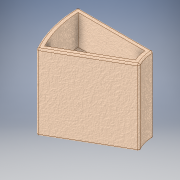
# Autodesk Inventor part: angular30
Saved by Autodesk Inventor 2019 (Build 230136000, 136)
## iProperties
Created: 2019-02-27
Part Number: angular30
Material: Concrete
Document SubType Name: Modeling
Designer: gaincarlo
Density: 2.40731 g/cm^3
Appearance: Exterior - Beige
Author: gaincarlo
Autodesk Inventor part; units mm, degrees
ref_plane "YZ Plane" through (0, 0, 0) normal (1, 0, 0) x (0, 1, 0)
ref_plane "XZ Plane" through (0, 0, 0) normal (0, 1, 0) x (-1, 0, 0)
ref_plane "XY Plane" through (0, 0, 0) normal (0, 0, 1) x (1, 0, 0)
sketch "Sketch1" plane through (0, 0, 0) normal (0, 1, 0) x (-1, 0, 0)
  line L0 (0, 0) -> (500, 0)
  arc A0 (500, 0) -> (399.5191, 375) centre (-250, 0) ccw
  arc A1 (0, 0) -> (-33.4936, 125) centre (-250, 0) ccw
  line L1 (-33.4936, 125) -> (399.5191, 375)
  line L2 (-404.937, 0) -> (679.6218, 0) projected
  dimension "d1" = 500
  dimension "d2" = 30
  dimension "d10" = 250
  constraints: 4 end point, 4 point on circle, 3 point on line, 2 centre point, 1 coincident, 1 horizontal
  measures "d1" distance of L0.start L0.end
  measures "d2" angle of L0 L1
  measures "d10" radius of A1
extrude "Extrusion1" add sketch "Sketch1" along normal blind 500
sketch "Sketch2" plane through (0, 500, 0) normal (0, 1, 0) x (1, 0, 0)
  arc A0 (0, 0) -> (33.4936, -125) centre (250, 0) ccw projected
  line L0 (33.4936, -125) -> (-399.5191, -375) projected
  arc A1 (-500, 0) -> (-399.5191, -375) centre (250, 0) ccw projected
  line L1 (-500, 0) -> (0, 0) projected
  line L2 (-387.9968, -333.7066) -> (-6.0913, -113.2133)
  arc A2 (-28.3882, -30) -> (-6.0913, -113.2133) centre (250, 0) ccw
  line L3 (-28.3882, -30) -> (-469.3747, -30)
  arc A3 (-469.3747, -30) -> (-387.9968, -333.7066) centre (250, 0) ccw
  dimension "d5" = 30
  constraints: 4 end point, 4 point on circle, 2 centre point, 3 other
  measures "d5" radial gap between concentric circles of A1 A3
extrude "Extrusion2" cut sketch "Sketch2" against normal blind 200 contours A3 L3 A2 L2
fillet "Fillet2" radius 10 12 edges at (-183.0127, 500, 250) (8.5185, 0, 64.7048) (0, 250, 0) (8.5185, 500, 64.7048) (33.4936, 250, 125) (-474.4444, 0, 194.1143) (-399.5191, 250, 375) (-474.4444, 500, 194.1143) (-500, 250, 0) (-250, 0, 0) (-250, 500, 0) (-183.0127, 0, 250)
body "Solid1"
